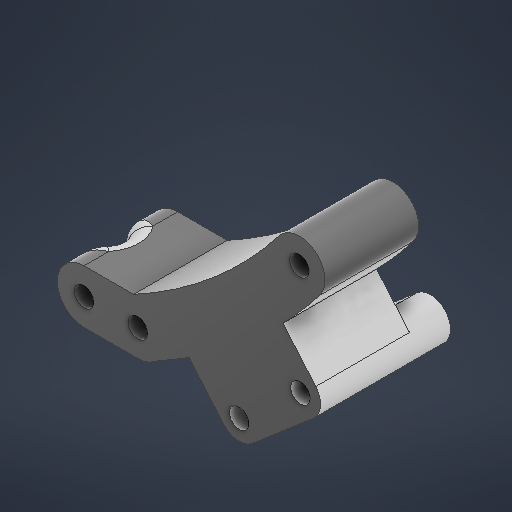
# Autodesk Inventor part: Lady Brown Ring Stop left
Saved by Autodesk Inventor 2025 (Build 290162000, 162)
## iProperties
Created: 2024-12-29
Part Number: Lady Brown Ring Stop left
Material: Generic
Document SubType Name: Modeling
Designer: Juan
Density: 1 g/cm^3
Appearance: Default
Author: Juan
Autodesk Inventor part; units mm, degrees
ref_plane "YZ Plane" through (0, 0, 0) normal (1, 0, 0) x (0, 1, 0)
ref_plane "XZ Plane" through (0, 0, 0) normal (0, 1, 0) x (-1, 0, 0)
ref_plane "XY Plane" through (0, 0, 0) normal (0, 0, 1) x (1, 0, 0)
sketch "Sketch1" plane through (0, 0, 0) normal (0, 0, 1) x (1, 0, 0)
  circle A0 centre (0, 0) radius 2.3241
  line L0 (0, 0) -> (12.7, 0) construction
  line L1 (0, -6.2992) -> (12.7, -6.2992)
  line L2 (12.7, 6.2992) -> (0, 6.2992)
  arc A1 (0, 6.2992) -> (0, -6.2992) centre (0, 0) ccw
  arc A2 (12.7, -6.2992) -> (12.7, 6.2992) centre (12.7, 0) ccw
  line L3 (12.7, 0) -> (50.8, 0)
  line L4 (50.8, 0) -> (50.8, 31.75)
  arc A3 (12.7, 0) -> (50.8, 31.75) centre (-39.6067, 101.5031) ccw
  line L5 (12.7, 0) -> (12.7, 6.2992)
  line L6 (12.7, -6.2992) -> (12.7, 0)
  arc A4 (12.7, 0) -> (50.8, 31.75) centre (-39.6067, 101.5031) ccw construction
  arc A5 (15.4698, -5.3749) -> (55.5873, 28.0564) centre (-39.6067, 101.5031) ccw
  arc A6 (9.9302, 5.3749) -> (46.0127, 35.4436) centre (-39.6067, 101.5031) ccw
  arc A7 (9.9302, 5.3749) -> (15.4698, -5.3749) centre (12.7, 0) ccw
  arc A8 (55.5873, 28.0564) -> (46.0127, 35.4436) centre (50.8, 31.75) ccw
  circle A9 centre (12.7, 0) radius 2.3241
  circle A10 centre (50.8, 31.75) radius 2.3241
  point P0 (6.35, 0)
  point P1 (17.0744, -4.5326)
  point P2 (11.6843, 6.2992)
  dimension "d0" = 4.6482
  dimension "d1" = 12.7
  dimension "d2" = 12.5984
  dimension "d3" = 38.1
  dimension "d4" = 31.75
  dimension "d5" = 4.6482
  dimension "d9" = 4.6482
  constraints: 16 end point, 16 point on circle, 11 centre point, 8 tangent, 3 coincident, 2 equal length, 2 horizontal, 2 perpendicular, 1 concentric, 1 midpoint
  measures "d0" diameter of A0
  measures "d1" distance of L0.start L0.end
  measures "d2" diameter of A2
  measures "d3" distance of L0.end L3.end
  measures "d4" distance of L3.end L4.end
  measures "d5" diameter of A9
  measures "d9" diameter of A10
extrude "Extrusion1" add sketch "Sketch1" along normal blind 22.098 contours A1 L2 A6 A7 L6 L1 | L6 A7 A5 A2 | A5 A7 L6 A9 L3 A2 | A2 L3 A5 | A7 A6 L2 L5 A9 L6 | A6 A8 A5 L4 A10 A3 A2 L2 | L3 A9 A3 A2 | A2 A3 A10 L4 A5 L3 | A2 A3 A9 L5 | A10 L4 A3 | A3 L4 A10
fillet "Fillet1" radius 25.4 1 edges at (17.0744, -4.5326, 11.049)
extrude "Extrusion2" cut sketch "Sketch1" along normal through all contours A10 L4 A3 | A3 L4 A10
sketch "Sketch2" plane through (0, -6.2992, 0) normal (0, -1, 0) x (1, 0, 0)
  line L0 (0, 0) -> (12.7, 0) projected
  line L1 (12.7, 0) -> (12.7, 22.098) projected
  line L2 (0, 22.098) -> (12.7, 22.098) projected
  line L3 (0, 0) -> (0, 22.098) projected
  line L4 (-2.3241, 0) -> (2.3241, 0) projected
  line L5 (-2.3241, 0) -> (-2.3241, 22.098)
  line L6 (0, 22.098) -> (-6.2992, 22.098) projected
  line L7 (0, 22.098) -> (-2.3241, 22.098)
  line L8 (-2.3241, 0) -> (-2.3241, 11.049)
  line L9 (-2.3241, 11.049) -> (-3.1178, 11.049)
  line L10 (-3.1178, 11.049) -> (-3.1496, 22.098)
  line L11 (-3.1178, 11.049) -> (-3.1496, 0)
  line L12 (0, 0) -> (-6.2992, 0) projected
  line L13 (-6.2992, 0) -> (-6.2992, 22.098) projected
  circle A0 centre (-6.2992, 11.049) radius 3.1814
  dimension "d12" = 0.7937
  constraints: 12 end point, 4 midpoint, 1 collinear, 1 horizontal alignment, 1 perpendicular, 1 point on line, 1 vertical, 2 other
  measures "d12" distance of L8.end L9.end
hole "Hole1" at (-6.2992, -6.2992, 11.049) direction (0, 1, 0) diameter 7.874 end through all
fillet "Fillet2" radius 4.2333 1 edges at (-6.2992, -0.0052, 14.986)
sketch "Sketch3" plane through (0, 0, 22.098) normal (0, 0, 1) x (1, 0, 0)
  circle A0 centre (50.8, 31.75) radius 4.7625
  circle A1 centre (12.7, 0) radius 4.7625
  circle A2 centre (0, 0) radius 4.7625
  arc A3 (35.202, -4.9015) -> (37.9881, -8.1507) centre (36.5951, -6.5261) ccw
  arc A4 (52.4497, 4.2495) -> (49.6636, 7.4987) centre (51.0566, 5.8741) ccw
  circle A5 centre (50.8, 31.75) radius 2.3241 projected
  circle A6 centre (50.8, 31.75) radius 2.3241 projected
  arc A7 (55.5873, 28.0564) -> (46.0127, 35.4436) centre (50.8, 31.75) ccw projected
  arc A8 (11.6843, 6.2992) -> (46.0127, 35.4436) centre (-39.6067, 101.5031) ccw projected
  line L0 (11.6843, 6.2992) -> (0, 6.2992) projected
  arc A9 (0, 6.2992) -> (0, -6.2992) centre (0, 0) ccw projected
  line L1 (0, -6.2992) -> (12.7, -6.2992) projected
  arc A10 (12.7, -6.2992) -> (16.3529, -5.1319) centre (12.7, 0) ccw projected
  arc A11 (18.7534, -3.6179) -> (16.3529, -5.1319) centre (31.0822, -25.8251) ccw projected
  arc A12 (18.7534, -3.6179) -> (55.5873, 28.0564) centre (-39.6067, 101.5031) ccw projected
  circle A13 centre (12.7, 0) radius 2.3241 projected
  circle A14 centre (0, 0) radius 2.3241 projected
  circle A15 centre (36.5951, -6.5261) radius 2.3241
  circle A16 centre (51.0566, 5.8741) radius 2.3241
  line L2 (51.0566, 5.8741) -> (36.5951, -6.5261) construction
  line L3 (47.9566, 9.4895) -> (33.495, -2.9107)
  line L4 (39.6951, -10.1415) -> (54.1567, 2.2587)
  arc A17 (54.1567, 2.2587) -> (47.9566, 9.4895) centre (51.0566, 5.8741) ccw
  arc A18 (33.495, -2.9107) -> (39.6951, -10.1415) centre (36.5951, -6.5261) ccw
  line L5 (32.9797, -9.6262) -> (24.7661, -0.0472)
  line L6 (54.672, 8.9742) -> (46.9177, 18.0175)
  point P0 (43.8258, -0.326)
  dimension "d21" = 4.6482
  dimension "d22" = 4.6482
  dimension "d23" = 9.525
  constraints: 12 end point, 12 point on circle, 9 centre point, 6 tangent, 2 coincident, 2 parallel, 1 midpoint, 2 other
  measures "d21" diameter of A15
  measures "d22" diameter of A16
  measures "d23" diameter of A18
extrude "Extrusion3" add sketch "Sketch3" against normal up to surface (22.098 mm away) contours L6 A17 L3 A18 L5 A12
extrude "Extrusion4" add sketch "Sketch3" against normal blind 30.6578 contours A17 L4 A18 L3
body "Solid1"
